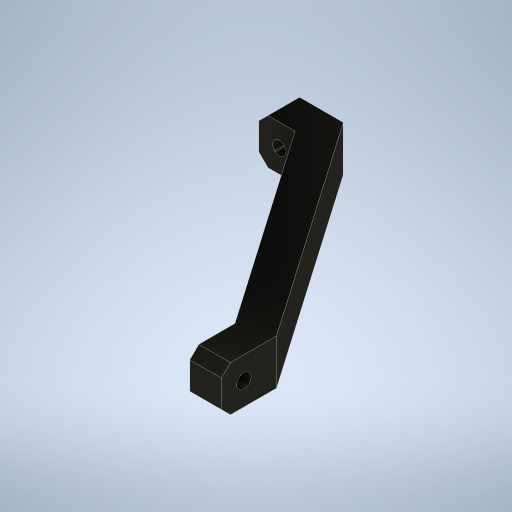
# Autodesk Inventor part: HoldingArms
Saved by Autodesk Inventor 2024.3 (Build 283343000, 343)
## iProperties
Created: 2025-01-30
Part Number: HoldingArms
Material: Generic
Document SubType Name: Modeling
Designer: migue
Density: 1 g/cm^3
Appearance: Gunmetal
Author: migue
Autodesk Inventor part; units mm, degrees
ref_plane "YZ Plane" through (0, 0, 0) normal (1, 0, 0) x (0, 1, 0)
ref_plane "XZ Plane" through (0, 0, 0) normal (0, 1, 0) x (-1, 0, 0)
ref_plane "XY Plane" through (0, 0, 0) normal (0, 0, 1) x (1, 0, 0)
sketch "Sketch1" plane through (0, 0, 0) normal (0, 1, 0) x (-1, 0, 0)
  line L0 (0, 0) -> (7, 0)
  line L1 (7, 0) -> (7, -10)
  line L2 (7, -10) -> (0, -10)
  line L3 (0, -10) -> (0, 0)
  line L4 (37.208, -60.52) -> (45.208, -60.52)
  line L5 (45.208, -60.52) -> (45.208, -53.52)
  line L6 (45.208, -53.52) -> (37.208, -53.52)
  line L7 (37.208, -53.52) -> (37.208, -60.52)
  line L8 (37.208, -53.52) -> (7, -10)
  line L9 (31.4575, -57.5115) -> (1.2495, -13.9915)
  line L10 (1.2495, -13.9915) -> (0, -12.1913)
  line L11 (0, -12.1913) -> (0, -10)
  line L12 (31.4575, -57.5115) -> (33.5458, -60.52)
  line L13 (33.5458, -60.52) -> (37.208, -60.52)
  dimension "d0" = 10
  dimension "d1" = 7
  dimension "d7" = 30.208
  dimension "d14" = 50.52
  dimension "d15" = 7
  dimension "d16" = 8
  dimension "d17" = 7
  constraints: 28 end point, 5 parallel, 3 perpendicular, 2 horizontal, 1 vertical
  measures "d0" distance of L2.end L0.start
  measures "d1" distance of L0.start L0.end
  measures "d7" distance from line of L1 L4.start
  measures "d14" distance from line of L2 L4.start
  measures "d15" distance of L4.end L5.end
  measures "d16" distance of L4.start L4.end
  measures "d17" distance between parallel lines of L8 L9
extrude "Extrusion1" add sketch "Sketch1" along normal blind 10
chamfer "Chamfer1" distance 2 angle 45 4 edges at (-45.208, 0, -57.02) (-45.208, 10, -57.02) (-3.5, 10, 0) (-3.5, 0, 0)
sketch "Sketch2" plane through (0, 0, -12.1913) normal (1, 0, 0) x (0, 0, -1)
  line L0 (-12.1913, 0) -> (-2.1913, 0) construction
  line L1 (-2.1913, 0) -> (-2.1913, 10) construction
  line L2 (-2.1913, 10) -> (-12.1913, 10) construction
  line L3 (-12.1913, 10) -> (-12.1913, 0) construction
  line L4 (-2.1913, 10) -> (-12.1913, 0) construction
  circle A0 centre (-7.1913, 5) radius 1.6
  dimension "d21" = 10
  dimension "d22" = 10
  dimension "d23" = 3.2
  constraints: 10 end point, 2 parallel, 1 centre point, 1 horizontal, 1 midpoint, 1 perpendicular
  measures "d21" distance of L2.end L1.end
  measures "d22" distance of L1.end L0.end
  measures "d23" diameter of A0
extrude "Extrusion2" cut sketch "Sketch2" against normal through all
sketch "Sketch3" plane through (-37.208, 0, -53.52) normal (0, 0, 1) x (1, 0, 0)
  line L0 (0, 0) -> (0, 10) projected
  line L1 (0, 10) -> (-10, 0) construction
  line L2 (0, 10) -> (14.1421, 10) construction
  line L3 (0, 5) -> (-3.5, 5)
  circle A0 centre (-3.5, 5) radius 1.5
  point P0 (37.208, 0)
  dimension "d26" = 135
  dimension "d27" = 3.5
  dimension "d28" = 3
  constraints: 6 end point, 2 horizontal, 1 centre point, 1 coincident, 1 equal length, 1 midpoint
  measures "d26" angle of L1 L2
  measures "d27" distance of L3.start L3.end
  measures "d28" diameter of A0
extrude "Extrusion3" cut sketch "Sketch3" against normal blind 10
body "Solid1"
